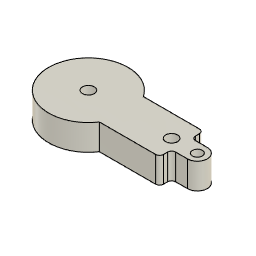
Webcam holder arm R (Autodesk Fusion 360 design; units mm, degrees)
Autodesk Fusion 360 part; units mm, degrees
sketch "Sketch1" plane through (0, 0, 0) normal (0, 0, 1) x (1, 0, 0)
  circle A0 centre (0, 0) radius 10
  constraint coincident A0.centre origin
extrude "Extrude1" add sketch "Sketch1" along normal blind 6.5
sketch "Sketch2" plane through (0, 0, 0) normal (0, 0, -1) x (1, 0, 0)
  circle A0 centre (0, 0) radius 10
  line L0 (0, 2.5) -> (30, 2.5)
  line L1 (30, 2.5) -> (30, -2.5)
  line L2 (30, -2.5) -> (0, -2.5)
  line L3 (0, -2.5) -> (0, 2.5)
  line L4 (0, 2.5) -> (30, -2.5) construction
  line L5 (30, 2.5) -> (0, -2.5) construction
  line L6 (15, 0) -> (0, 0) construction
  point P0 (15, 0)
  dimension "d19" = 5
  dimension "d20" = 30
  constraint horizontal L0
  constraint perpendicular L0 L1
  constraint parallel L0 L2
  constraint parallel L1 L3
  constraint coincident L4 P0
  constraint coincident L5 P0
  constraint midpoint L4 P0
  constraint coincident P0 L6.start
  constraint coincident A0.centre L6.end
  constraint horizontal L6
  constraint coincident A0.centre L3
  measures "d19" distance of L0.end L1.end
  measures "d20" distance of L1.end L2.end
extrude "Extrude2" add sketch "Sketch2" against normal up to surface (6.5 mm away) contours A0 L0 L1 L2
hole "Hole1" at (0, 0, 6.5) direction (0, 0, -1) diameter 3 end through all
fillet "Fillet1" radius 2.5 2 edges at (30, -2.5, 3.25) (30, 2.5, 3.25)
hole "Hole2" at (27.5, 0, 6.5) direction (0, 0, -1) diameter 2.5 end through all
sketch "Sketch4" plane through (0, 0, 0) normal (0, 0, -1) x (1, 0, 0)
  circle A0 centre (27.5, 0) radius 1.25
  circle A1 centre (0, 0) radius 1.5
  arc A2 (27.5, -2.5) -> (27.5, 2.5) centre (27.5, 0) ccw
  line L0 (27.5, 2.5) -> (9.6825, 2.5)
  arc A3 (9.6825, 2.5) -> (9.6825, -2.5) centre (0, 0) ccw
  line L1 (9.6825, -2.5) -> (27.5, -2.5)
  line L2 (1.5, 5.546) -> (23.5, 5.546)
  line L3 (23.5, 5.546) -> (23.5, -5.546)
  line L4 (23.5, -5.546) -> (1.5, -5.546)
  line L5 (1.5, -5.546) -> (1.5, 5.546)
  line L6 (1.5, 5.546) -> (23.5, -5.546) construction
  line L7 (23.5, 5.546) -> (1.5, -5.546) construction
  line L8 (12.5, 0) -> (23.5, 0) construction
  point P0 (12.5, 0)
  dimension "d35" = 4
  constraint horizontal L2
  constraint perpendicular L2 L3
  constraint parallel L2 L4
  constraint parallel L3 L5
  constraint coincident L6 P0
  constraint coincident L7 P0
  constraint coincident P0 L8.start
  constraint midpoint L3 L8.end
  constraint tangent A1 L5
  measures "d35" distance of A0.centre L3
extrude "Extrude4" add sketch "Sketch4" against normal up to surface (6.5 mm away) contours A3 L1 L3 L4 | L0 A3 L2 L3
sketch "Sketch6" plane through (0, 0, 6.5) normal (0, 0, 1) x (-1, 0, 0)
  line L0 (-23.5, 5.546) -> (-23.5, 2.5)
  line L1 (-23.5, 2.5) -> (-27.5, 2.5)
  arc A0 (-27.5, 2.5) -> (-27.5, -2.5) centre (-27.5, 0) ccw
  line L2 (-27.5, -2.5) -> (-23.5, -2.5)
  line L3 (-23.5, -2.5) -> (-23.5, -5.546)
  line L4 (-23.5, -5.546) -> (-8.3212, -5.546)
  arc A1 (-8.3212, -5.546) -> (-8.3212, 5.546) centre (0, 0) ccw
  line L5 (-8.3212, 5.546) -> (-23.5, 5.546)
  circle A2 centre (-27.5, 0) radius 1.25
  circle A3 centre (0, 0) radius 1.5
  circle A4 centre (-21, 0) radius 1
  dimension "d36" = 2.5
  measures "d36" distance of L0 A4.centre
fillet "Fillet2" radius 1 4 edges at (23.5, 5.546, 3.25) (23.5, -5.546, 3.25) (23.5, 2.5, 3.25) (23.5, -2.5, 3.25)
hole "Hole4" at (21, 0, 6.5) direction (0, 0, -1) diameter 3 end through all
